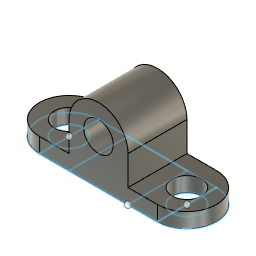
A4 (Autodesk Fusion 360 design; units mm, degrees)
Autodesk Fusion 360 part; units mm, degrees
sketch "Sketch1" plane through (0, 0, 0) normal (1, 0, 0) x (0, 1, 0)
sketch "Sketch2" plane through (0, 0, 0) normal (0, 0, 1) x (1, 0, 0)
  line L0 (-30, 20) -> (50, 20)
  line L1 (50, 20) -> (50, -20)
  line L2 (50, -20) -> (-30, -20)
  line L3 (-30, -20) -> (-30, 20)
  line L4 (-30, -20) -> (-10, -20)
  line L5 (50, -20) -> (30, -20)
  line L6 (-10, -20) -> (30, -20)
  line L7 (30, -20) -> (30, 20)
  line L8 (30, 20) -> (-10, 20)
  line L9 (-10, 20) -> (-10, -20)
  arc A0 (-30, 20) -> (-30, -20) centre (-30, 0) ccw
  line L10 (50, 20) -> (50, -20)
  arc A1 (50, -20) -> (50, 20) centre (50, 0) ccw
  circle A2 centre (-30, 0) radius 10
  circle A3 centre (50, 0) radius 10
  dimension "d1" = 80
  dimension "d2" = 40
  dimension "d3" = 20
  dimension "d4" = 20
  dimension "d5" = 20
  dimension "d6" = 20
  constraint horizontal L0
  constraint vertical L1
  constraint horizontal L2
  constraint vertical L3
  constraint perpendicular L3 L4
  constraint perpendicular L1 L5
  constraint horizontal L6
  constraint vertical L7
  constraint horizontal L8
  constraint vertical L9
  constraint coincident L0 L7.end
  constraint tangent L0 A0
  constraint tangent L0 A1
  constraint concentric A0 A2
  constraint concentric A1 A3
  measures "d1" distance of L0.start L0.end
  measures "d2" distance of L0.start L2.end
  measures "d3" distance of L2.end L4.end
  measures "d4" distance of L1.end L5.end
  measures "d5" diameter of A2
  measures "d6" diameter of A3
extrude "Extrude2" add sketch "Sketch2" along normal blind 30 contours L0 L2 L6 L7 L8 L9 makes body 1
extrude "Extrude1" add sketch "Sketch2" along normal blind 10 separate body contours L0 L2 L3 L4 L9 A2 | L3 A0 A2 | L0 L1 L2 L5 L7 L10 A3 | L1 L10 A1 A3 makes body 2 at (-13.3333, 0, 0) makes body 3 at (33.3333, 0, 10)
sketch "Sketch3" plane through (0, 0, 0) normal (0, 1, 0) x (1, 0, 0)
  circle A0 centre (10, -30) radius 20
extrude "Extrude3" add sketch "Sketch3" along normal blind 20 and the other way blind 20 bodies 1
hole "Hole1" at (10, -20, 30) direction (0, 1, 0) diameter 20 depth 40 tip angle 180 bodies 1
combine "Combine1" operation add target body 1 tool bodies 3 2
named bodies: "A4"
